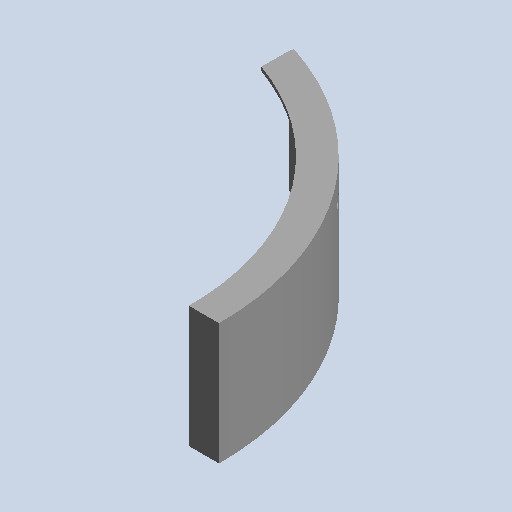
# Autodesk Inventor part: Bottom_Enclosure_2
Saved by Autodesk Inventor 2026 (Build 300175050, 175E)
## iProperties
Part Number: Bottom_Enclosure_2
Material: Generic
Document SubType Name: Modeling
Designer: Kartik
Mass: 96.5252 g
Surface Area: 667.691 cm^2
Volume: 96.5252 cm^3
Density: 1 g/cm^3
Appearance: Default
Author: Kartik
Autodesk Inventor part; units mm, degrees
ref_plane "YZ Plane" through (0, 0, 0) normal (1, 0, 0) x (0, 1, 0)
ref_plane "XZ Plane" through (0, 0, 0) normal (0, 1, 0) x (-1, 0, 0)
sketch "Sketch1" plane through (0, 0, 0) normal (0, 1, 0) x (-1, 0, 0)
  arc A0 (-220, 0) -> (-67, -209.5495) centre (0, 0) ccw
  arc A1 (-217, 0) -> (-67, -206.3977) centre (0, 0) ccw
  line L0 (-220, 0) -> (-217, 0)
  line L1 (0, -220) -> (0, -217)
  line L2 (0, -220) -> (-67, -220)
  line L3 (0, -220) -> (67, -220) construction
  line L4 (-67, -220) -> (-67, -206.3977)
  line L5 (-67, -206.3977) -> (-65.0308, -207.0265)
  line L6 (-67, -206.3977) -> (-68.4601, -210.9695)
  point P0 (-67.9127, -209.2555)
  dimension "d0" = 440
  dimension "d1" = 3
  dimension "d2" = 67
  dimension "d3" = 180
  dimension "d9" = 90
  constraints: 14 end point, 4 point on circle, 3 horizontal, 2 centre point, 2 perpendicular, 1 coincident, 1 collinear, 1 point on line
  measures "d0" diameter of A0
  measures "d1" radial gap between concentric circles of A0 A1
  measures "d2" distance of L1.start L2.end
  measures "d3" angle of L2 L3
  measures "d9" angle of L5 L6
extrude "Extrusion1" add sketch "Sketch1" along normal blind 92.5 contours L0 A1 L6 A0
sketch "Sketch3" plane through (0, 92.5, 0) normal (0, 1, 0) x (1, 0, 0)
  arc A0 (217, 0) -> (67, 206.3977) centre (0, 0) ccw projected
  arc A1 (197, 0) -> (60.8249, 187.3748) centre (0, 0) ccw
  line L0 (60.8249, 187.3748) -> (67, 206.3977)
  line L1 (197, 0) -> (217, 0)
  dimension "d10" = 20
  constraints: 4 end point, 3 point on circle, 1 centre point, 1 horizontal
  measures "d10" radial gap between concentric circles of A0 A1
extrude "Extrusion3" add sketch "Sketch3" against normal blind 3
sketch "Sketch4" plane through (0, 92.5, 0) normal (0, 1, 0) x (1, 0, 0)
  line L0 (197, 0) -> (220, 0) projected
  arc A0 (197, 0) -> (60.8249, 187.3748) centre (0, 0) ccw projected
  arc A1 (220, 0) -> (67.9127, 209.2555) centre (0, 0) ccw projected
  line L1 (196.9772, 3) -> (219.9795, 3)
  dimension "d13" = 3
  constraints: 2 end point, 2 point on circle, 1 horizontal
  measures "d13" distance between parallel lines of L0 L1
extrude "Extrusion4" add sketch "Sketch4" against normal up to surface (92.5 mm away)
sketch "Sketch5" plane through (0, 89.5, 0) normal (0, -1, 0) x (1, 0, 0)
  arc A0 (60.8249, -187.3748) -> (196.9772, -3) centre (0, 0) ccw projected
  line L0 (60.8249, -187.3748) -> (67, -206.3977) projected
  arc A1 (67, -206.3977) -> (216.9793, -3) centre (0, 0) ccw projected
  line L1 (67, -206.3977) -> (67, -185.2566)
  line L2 (67, -206.3977) -> (88.1411, -206.3977) construction
  dimension "d16" = 90
  constraints: 4 end point, 1 horizontal, 1 perpendicular, 1 point on circle
  measures "d16" angle of L2 L1
extrude "Extrusion5" cut sketch "Sketch5" against normal through all
sketch "Sketch6" plane through (0, 0, 0) normal (0, -1, 0) x (1, 0, 0)
  line L0 (0, 0) -> (155.5635, -155.5635)
  arc A0 (67.9127, -209.2555) -> (220, 0) centre (0, 0) ccw projected
  line L1 (0, 0) -> (220, 0) construction
  dimension "d19" = 45
  constraints: 4 end point, 1 equal length, 1 horizontal, 1 point on circle
  measures "d19" angle of L0 L1
ref_plane "Work Plane1" through (155.5635, 0, -155.5635) normal (0.7071, 0, -0.7071) x (0, 1, 0)
sketch "Sketch7" plane through (155.5635, 0, -155.5635) normal (0.7071, 0, -0.7071) x (0, 1, 0)
  circle A0 centre (72.5, -12.5) radius 5
  circle A1 centre (72.5, 12.5) radius 5
  line L0 (92.5, -99.9445) -> (92.5, 155.5635) projected
  line L1 (0, 0) -> (103.0589, 0)
  dimension "d20" = 10
  dimension "d21" = 10
  dimension "d22" = 25
  dimension "d23" = 20
  dimension "d24" = 20
  dimension "d25" = 12.5
  constraints: 2 centre point, 2 end point, 1 perpendicular
  measures "d20" diameter of A0
  measures "d21" diameter of A1
  measures "d22" distance of A1.centre A0.centre
  measures "d23" distance from line of L0 A0.centre
  measures "d24" distance from line of L0 A1.centre
  measures "d25" distance from line of L1 A0.centre
extrude "Extrusion6" cut sketch "Sketch7" against normal through all
body "Solid1"
